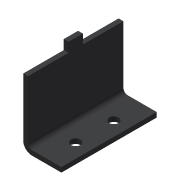
# Autodesk Inventor part: XBRACKET
Saved by Autodesk Inventor 2022 Beta2 (Build 260130000, 130) ContinuousBuild 0
## iProperties
Shininess: 64.0
Length Units: 11272
Angle Units: 11279
Time Units: 11290
Mass Units: 11286
Length Display Precision: 3
Angle Display Precision: 2
Compacted: True
Part Number: XBRACKET
Document SubType Name: Modeling
Created: 2004-02-26
Designer: mpaknia
Manufacturer: Standard
Standards Organization: Custom
Density: 1 g/cm^3
Material: Generic
Appearance: Generic
Density: 0.0
Volumn: 0.0
Area: 0.0
PropertySet Name: Model Information
Control State: 0
Master: False
Checked Out: False
Author: mpaknia
Autodesk Inventor part; units mm, degrees
ref_plane "YZ Plane" through (0, 0, 0) normal (1, 0, 0) x (0, 1, 0)
ref_plane "XZ Plane" through (0, 0, 0) normal (0, 1, 0) x (-1, 0, 0)
ref_plane "XY Plane" through (0, 0, 0) normal (0, 0, 1) x (1, 0, 0)
sketch "Sketch1" plane through (0, 0, 0) normal (0, 0, 1) x (1, 0, 0)
  line L0 (0, 232.5603) -> (0, -22.9879) projected
  line L1 (-15.3679, 0) -> (133.5003, 0) projected
  line L2 (0, 177.8) -> (0, 22.86)
  line L3 (22.86, 0) -> (101.6, 0)
  line L4 (101.6, 0) -> (101.6, 12.7)
  line L5 (101.6, 12.7) -> (24.13, 12.7)
  line L6 (12.7, 24.13) -> (12.7, 177.8)
  line L7 (12.7, 177.8) -> (0, 177.8)
  arc A0 (0, 22.86) -> (22.86, 0) centre (22.86, 22.86) ccw
  arc A1 (12.7, 24.13) -> (24.13, 12.7) centre (24.13, 24.13) ccw
  dimension "d0" = 22.86
  dimension "d1" = 12.7
  dimension "d2" = 177.8
  dimension "d4" = 12.7
  dimension "d6" = 101.6
  dimension "d7" = 11.43
  constraints: 12 end point, 4 parallel, 4 point on circle, 4 tangent, 2 centre point, 2 collinear, 2 perpendicular
  measures "d0" radius of A0
  measures "d1" distance of L6.end L2.start
  measures "d2" distance between parallel lines of L1 L7
  measures "d4" distance between parallel lines of L3 L5
  measures "d6" distance between parallel lines of L2 L4
  measures "d7" radius of A1
extrude "Extrusion1" add sketch "Sketch1" against normal blind 254 contours L7 L6 A1 L5 L4 L1 A0 L0
sketch "Sketch2" plane through (24.13, 12.7, 0) normal (0, 1, 0) x (1, 0, 0)
  line L0 (77.47, 0) -> (0, 0) projected
  line L1 (77.47, 0) -> (77.47, 254) projected
  point P0 (39.37, 76.2)
  dimension "d10" = 38.1
  dimension "d11" = 76.2
  measures "d10" distance from line of L1 point (39.37, 76.2)
  measures "d11" distance from line of L0 point (39.37, 76.2)
hole "Hole1" at (63.5, 12.7, -76.2) direction (0, -1, 0) diameter 25.4 end through all
pattern_linear "Rectangular Pattern1" count 2 spacing 101.6 along (0, 0, -1) of "Hole1"
sketch "Sketch3" plane through (12.7, 24.13, 0) normal (1, 0, 0) x (0, 0, -1)
  line L0 (0, 153.67) -> (254, 153.67) projected
  line L1 (0, 0) -> (0, 153.67) projected
  line L2 (0, 0) -> (254, 0) projected
  line L3 (107.95, 153.67) -> (107.95, 179.07)
  line L4 (107.95, 179.07) -> (146.05, 179.07)
  line L5 (146.05, 179.07) -> (146.05, 153.67)
  dimension "d22" = 25.4
  dimension "d23" = 38.1
  dimension "d24" = 107.95
  constraints: 6 end point, 3 perpendicular, 2 point on line
  measures "d22" distance of L4.end L5.end
  measures "d23" distance of L3.end L4.end
  measures "d24" distance between parallel lines of L1 L3
extrude "Extrusion2" add sketch "Sketch3" against normal blind 12.7
body "Solid1"
